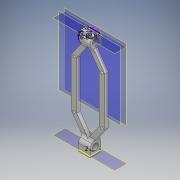
# Autodesk Inventor part: mousetrapMount
Saved by Autodesk Inventor 2018 (Build 220112000, 112)
## iProperties
Created: 2018-11-24
Part Number: mousetrapMount
Material: Generic
Document SubType Name: Modeling
Designer: Prakash
Density: 1 g/cm^3
Appearance: Default
Author: Prakash
Autodesk Inventor part; units mm, degrees
ref_plane "YZ Plane" through (0, 0, 0) normal (1, 0, 0) x (0, 1, 0)
ref_plane "XY Plane" through (0, 0, 0) normal (0, 0, 1) x (1, 0, 0)
sketch "Sketch3" plane through (0, 0, 0) normal (1, 0, 0) x (0, 1, 0)
  circle A0 centre (0, 0) radius 5.4
  circle A1 centre (0, 0) radius 9.4
  dimension "d0" = 10.8
  dimension "d1" = 18.8
  constraints: 2 centre point, 2 coincident
  measures "d0" diameter of A0
  measures "d1" diameter of A1
extrude "Extrusion1" add sketch "Sketch3" along normal blind 20
ref_plane "Work Plane1" through (0, 9.4, 0) normal (0, 1, 0) x (-1, 0, 0)
sketch "Sketch4" plane through (0, 9.4, 0) normal (0, 1, 0) x (-1, 0, 0)
  line L0 (-20, 9.4) -> (-20, -9.4) projected
  line L1 (-20, 0) -> (0, 0) construction
  line L2 (0, 9.4) -> (-20, 9.4) projected
  line L3 (-20, 9.4) -> (-20, -9.4) projected
  line L4 (0, -9.4) -> (0, 9.4) projected
  line L5 (0, -9.4) -> (-20, -9.4) construction
  line L6 (-59.213, -14.95) -> (39.213, -14.95) construction
  line L7 (39.213, -14.95) -> (39.213, -59.4) construction
  line L8 (39.213, -59.4) -> (-59.213, -59.4) construction
  line L9 (-59.213, -59.4) -> (-59.213, -14.95) construction
  line L10 (-59.213, -14.95) -> (39.213, -59.4) construction
  line L11 (39.213, -14.95) -> (-59.213, -59.4) construction
  line L12 (-59.213, -59.4) -> (39.213, -59.4) construction
  line L13 (39.213, -59.4) -> (39.213, -103.85) construction
  line L14 (39.213, -103.85) -> (-59.213, -103.85) construction
  line L15 (-59.213, -103.85) -> (-59.213, -59.4) construction
  line L16 (-59.213, -59.4) -> (39.213, -103.85) construction
  line L17 (39.213, -59.4) -> (-59.213, -103.85) construction
  line L18 (-10, -37.175) -> (-59.213, -37.175) construction
  line L19 (-10, -37.175) -> (39.213, -37.175) construction
  line L20 (-10, -81.625) -> (-59.213, -81.625) construction
  line L21 (-10, -81.625) -> (39.213, -81.625) construction
  line L22 (-20, -9.4) -> (-39.6065, -37.175)
  line L23 (-10, -9.4) -> (-29.6065, -37.175)
  line L24 (-39.6065, -37.175) -> (-39.6065, -59.4)
  line L25 (-10, -9.4) -> (9.6065, -37.175)
  line L26 (0, -9.4) -> (19.6065, -37.175)
  line L27 (19.6065, -37.175) -> (19.6065, -59.4)
  line L28 (-34.6065, -37.175) -> (-34.6065, -81.625) construction
  line L29 (14.6065, -81.625) -> (14.6065, -37.175) construction
  line L30 (-29.6065, -37.175) -> (-29.6065, -59.4)
  line L31 (9.6065, -37.175) -> (9.6065, -59.4)
  line L32 (-39.6065, -59.4) -> (-29.6065, -59.4)
  line L33 (9.6065, -59.4) -> (19.6065, -59.4)
  line L34 (-20, -9.4) -> (-10, -9.4)
  line L35 (0, -9.4) -> (-20, -9.4) projected
  line L36 (-10, -9.4) -> (0, -9.4)
  point P0 (-10, 0)
  dimension "d5" = 44.45
  dimension "d6" = 49.213
  dimension "d7" = 44.45
  dimension "d21" = 50
  constraints: 62 end point, 15 midpoint, 10 point on line, 8 parallel, 5 perpendicular, 3 horizontal, 2 collinear, 2 vertical, 1 equal length, 2 other
  measures "d5" distance of L6.end L7.end
  measures "d6" distance from line of L7 L18.start
  measures "d7" distance of L12.end L13.end
  measures "d21" distance between parallel lines of L8 L5
ref_plane "Work Plane2" through (0, 0, 0) normal (0, 1, 0) x (-1, 0, 0)
sketch "Sketch5" plane through (0, 0, 0) normal (0, 1, 0) x (-1, 0, 0)
  line L0 (-20, -9.4) -> (-39.6065, -37.175) projected
  line L1 (-10, -9.4) -> (-29.6065, -37.175) projected
  line L2 (-10, -9.4) -> (9.6065, -37.175) projected
  line L3 (0, -9.4) -> (19.6065, -37.175) projected
  line L4 (19.6065, -37.175) -> (19.6065, -59.4) projected
  line L5 (9.6065, -37.175) -> (9.6065, -59.4) projected
  line L6 (-29.6065, -37.175) -> (-29.6065, -59.4) projected
  line L7 (-39.6065, -37.175) -> (-39.6065, -59.4) projected
  line L8 (-39.6065, -59.4) -> (-29.6065, -59.4) projected
  line L9 (9.6065, -59.4) -> (19.6065, -59.4) projected
  line L10 (0, -9.4) -> (-20, -9.4) projected
  point P0 (0, 0)
  point P1 (-34.6065, -37.175)
  point P2 (14.6065, -37.175)
extrude "Extrusion2" add sketch "Sketch5" along normal mid plane 6
sketch "Sketch7" plane through (0, -3, 0) normal (0, -1, 0) x (1, 0, 0)
  point P0 (0, 0)
  point P1 (34.6065, -37.175)
  point P2 (-14.6065, -37.175)
hole "Hole1" at (-14.6065, -3, -37.175) at (34.6065, -3, -37.175) direction (0, 1, 0) diameter 4.305 end through all clearance for "Flat Head Machine Screw (82)" size "#6" standard "Ansi Unified Screw Threads"
sketch "Sketch8" plane through (0, 0, -9.4) normal (0, 0, 1) x (1, 0, 0)
  line L0 (0, 3) -> (10, 3) projected
  line L1 (20, 0) -> (20, -3) projected
  line L2 (0, 3) -> (20, 3)
  line L3 (20, 3) -> (20, -3)
  line L4 (20, -3) -> (0, -3)
  line L5 (0, -3) -> (0, 3)
  point P0 (0, 0)
  constraints: 8 end point, 2 parallel, 1 horizontal, 1 perpendicular
extrude "Extrusion4" add sketch "Sketch8" along normal up to surface
ref_plane "Work Plane3" through (0, 0, 9.25) normal (0, 0, -1) x (-1, 0, 0)
ref_plane "Work Plane5" through (0, 9.4, 0) normal (0, 1, 0) x (-1, 0, 0)
sketch "Sketch14" plane through (0, 9.4, 0) normal (0, 1, 0) x (-1, 0, 0)
  line L0 (-20, -8.9084) -> (0, -8.9084) projected
  line L1 (0, -8.9084) -> (0, -8.9084) projected
  line L2 (0, -8.9084) -> (-20, -8.9084) projected
  line L3 (-20, -8.9084) -> (-20, -8.9084) projected
  line L4 (-20, 9.4) -> (-20, -8.9084) projected
  line L5 (0, -8.9084) -> (0, 9.4) projected
  line L6 (-20, -8.9084) -> (0, 9.4) construction
  line L7 (-20, 9.4) -> (0, -8.9084) construction
  point P0 (0, 0)
  point P1 (-10, 0.2458)
  constraints: 4 end point, 1 midpoint
sketch "Sketch15" plane through (0, 9.4, 0) normal (0, 1, 0) x (-1, 0, 0)
  line L0 (-20, 9.4) -> (0, -8.9084) construction
  line L1 (-20, -8.9084) -> (0, 9.4) construction
  circle A0 centre (-10, 0.2458) radius 4
  point P0 (0, 0)
  dimension "d28" = 8
  constraints: 1 centre point, 1 coincident
  measures "d28" diameter of A0
extrude "Extrusion6" add sketch "Sketch15" against normal up to surface
extrude "Extrusion7" add sketch "Sketch15" along normal blind 1
sketch "Sketch16" plane through (10, 10.4, 0.2458) normal (0, 1, 0) x (1, 0, 0)
  line L0 (10, 9.1542) -> (-10, -9.1542) construction
  line L1 (10, -9.1542) -> (-10, 9.1542) construction
  circle A0 centre (0, 0) radius 4 projected
  circle A1 centre (0, 0) radius 2.5275
  point P0 (-10, 0.2458)
  dimension "d33" = 5.055
  constraints: 1 centre point, 1 coincident
  measures "d33" diameter of A1
extrude "Extrusion8" cut sketch "Sketch16" against normal blind 3.81 contours A1
sketch "Sketch17" plane through (10, 10.4, 0.2458) normal (0, 1, 0) x (1, 0, 0)
  line L0 (10, -9.1542) -> (-10, 9.1542) construction
  line L1 (10, 9.1542) -> (-10, -9.1542) construction
  circle A0 centre (0, 0) radius 2.6545
  point P0 (-10, 0.2458)
  dimension "d36" = 5.309
  constraints: 1 centre point, 1 coincident
  measures "d36" diameter of A0
loft "Loft1" cut profiles "Sketch17" section 1 edges at (7.4725, 6.59, 0.2458)
sketch "Sketch18" plane through (10, 6.59, 0.2458) normal (0, 1, 0) x (1, 0, 0)
  line L0 (10, -9.1542) -> (-10, 9.1542) construction
  line L1 (10, 9.1542) -> (-10, -9.1542) construction
  circle A0 centre (0, 0) radius 1.8
  point P0 (-10, 0.2458)
  dimension "d41" = 3.6
  constraints: 1 centre point, 1 coincident
  measures "d41" diameter of A0
extrude "Extrusion9" cut sketch "Sketch18" against normal up to surface
sketch "Sketch21" plane through (0, 0, 9.25) normal (0, 0, -1) x (-1, 0, 0)
  line L0 (-20, 9.4) -> (-20, -9.4) construction
  line L1 (0, -9.4) -> (0, 9.4) construction
  line L2 (0, -9.4) -> (-20, -9.4) construction
  line L3 (0, -9.4) -> (-20, -9.4)
  line L4 (-20, -9.4) -> (-20, 7.95)
  line L5 (-20, 7.95) -> (0, 7.95)
  line L6 (0, 7.95) -> (0, -9.4)
  point P0 (0, 0)
  point P1 (-13.9963, 9.25)
  point P2 (-6.0037, 9.25)
  point P3 (-20, 3)
  point P4 (-20, -3)
  point P5 (0, -3)
  point P6 (0, 3)
  point P7 (-13.9922, 9.25)
  point P8 (-6.0078, 9.25)
  point P9 (-13.9924, 9.375)
  point P10 (-6.0076, 9.375)
  dimension "d45" = 17.35
  constraints: 8 end point, 2 perpendicular, 2 point on line, 1 horizontal, 1 other
  measures "d45" distance between parallel lines of L2 L5
fillet "Fillet1" radius 8 2 edges at (10, 3, -8.9084) (10, -3, -8.9084)
sketch "Sketch23" plane through (39.6065, 3, -59.4) normal (0, 0, -1) x (-1, 0, 0)
  line L0 (10, -6) -> (10, 0) projected
  line L1 (0, 0) -> (10, 0) projected
  line L2 (0, -6) -> (0, 0) projected
  line L3 (10, -6) -> (0, -6) projected
  line L4 (59.213, -6) -> (59.213, 0) projected
  line L5 (49.213, 0) -> (59.213, 0) projected
  line L6 (49.213, -6) -> (49.213, 0) projected
  line L7 (59.213, -6) -> (49.213, -6) projected
  point P0 (39.6065, -3)
extrude "Extrusion11" add sketch "Sketch23" along normal blind 20
mirror "Mirror4" about plane through (-14.6065, 0, -79.4) normal (0, 0, -1) of "Extrusion1", "Hole1", "Extrusion4", "Extrusion6", "Extrusion7", "Extrusion8", "Loft1", "Extrusion9", "Fillet1", "Extrusion11", "Extrusion2"
sketch "Sketch24" plane through (0, 0, -168.05) normal (0, 0, 1) x (-1, 0, 0)
  line L0 (0, -9.4) -> (-20, -9.4) construction
  line L1 (-20, -9.4) -> (-20, 7.95) projected
  line L2 (-20, 7.95) -> (0, 7.95) projected
  line L3 (0, 7.95) -> (0, -9.4) projected
  line L4 (-20, 7.95) -> (-20, -9.4)
  line L5 (0, -9.4) -> (-20, -9.4)
  point P0 (0, 0)
  constraints: 4 end point, 1 collinear, 1 perpendicular
ref_plane "Work Plane8" through (0, 0, -168.2) normal (0, 0, -1) x (-1, 0, 0)
sketch "Sketch29" plane through (0, 0, -168.2) normal (0, 0, -1) x (-1, 0, 0)
  line L0 (0, -9.4) -> (-20, -9.4) construction
  line L1 (-20, 9.4) -> (-20, -9.4) construction
  line L2 (0, -9.4) -> (0, 9.4) construction
  line L3 (-20, 7.95) -> (0, 7.95) projected
  line L4 (-20, 7.95) -> (-20, -9.4)
  line L5 (-20, -9.4) -> (0, -9.4)
  line L6 (0, -9.4) -> (0, 7.95)
  point P0 (0, 0)
  constraints: 6 end point, 2 collinear, 1 perpendicular
extrude "Extrusion16" add sketch "Sketch29" against normal up to surface
sketch "Sketch30" plane through (0, 0, -168.2) normal (0, 0, -1) x (-1, 0, 0)
  line L0 (0, 7.95) -> (0, -9.4) projected
  line L1 (-20, 7.95) -> (0, 7.95) projected
  line L2 (-20, -9.4) -> (-20, 7.95) projected
  line L3 (0, -9.4) -> (-20, -9.4) projected
  line L4 (-20, 7.95) -> (0, -9.4) construction
  line L5 (0, 7.95) -> (-20, -9.4) construction
  circle A0 centre (-10, -0.725) radius 1
  point P0 (0, 0)
  dimension "d66" = 2
  constraints: 4 end point, 1 centre point, 1 midpoint
  measures "d66" diameter of A0
extrude "Extrusion17" cut sketch "Sketch30" against normal up to surface contours A0
extrude "Extrusion18" add sketch "Sketch30" along normal blind 3
ref_plane "Work Plane6" through (0, 0, -168.05) normal (0, 0, -1) x (-1, 0, 0)
ref_plane "Work Plane7" through (0, 9.4, -158.8) normal (0, -1, 0) x (-1, 0, 0)
equation "\"d7\" = d5"
body "Solid1"
